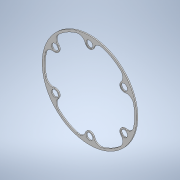
# Autodesk Inventor part: Bottom Lid
Saved by Autodesk Inventor 2020 (Build 240168000, 168)
## iProperties
Created: 2020-03-28
Part Number: Bottom Lid
Material: Generic
Document SubType Name: Modeling
Designer: pengpeng
Density: 1 g/cm^3
Appearance: Default
Author: pengpeng
Autodesk Inventor part; units mm, degrees
ref_plane "YZ Plane" through (0, 0, 0) normal (1, 0, 0) x (0, 1, 0)
ref_plane "XZ Plane" through (0, 0, 0) normal (0, 1, 0) x (-1, 0, 0)
ref_plane "XY Plane" through (0, 0, 0) normal (0, 0, 1) x (1, 0, 0)
sketch "Sketch1" plane through (0, 0, 0) normal (0, 0, 1) x (1, 0, 0)
  circle A0 centre (0, 0) radius 68
  circle A1 centre (0, 0) radius 65
  line L0 (0, 0) -> (0, 94.1006) construction
  line L1 (0, 0) -> (-100.1308, -57.8105) construction
  line L2 (0, 0) -> (108.5937, -62.6966) construction
  line L3 (0, 0) -> (0, -119.3862) construction
  line L4 (0, 0) -> (-99.0917, 57.2106) construction
  line L5 (0, 0) -> (100.283, 57.8984) construction
  circle A2 centre (0, 57.5) radius 4.8
  circle A3 centre (-49.7965, 28.75) radius 4.8
  circle A4 centre (-49.7965, -28.75) radius 4.8
  circle A5 centre (0, -57.5) radius 4.8
  circle A6 centre (49.7965, -28.75) radius 4.8
  circle A7 centre (49.7965, 28.75) radius 4.8
  circle A8 centre (0, 57.5) radius 6.3
  circle A9 centre (-49.7965, 28.75) radius 6.3
  circle A10 centre (-49.7965, -28.75) radius 6.3
  circle A11 centre (0, -57.5) radius 6.3
  circle A12 centre (49.7965, -28.75) radius 6.3
  circle A13 centre (49.7965, 28.75) radius 6.3
  circle A14 centre (-15.5907, 52.744) radius 10
  circle A15 centre (15.5907, 52.744) radius 10
  circle A16 centre (-53.473, 12.87) radius 10
  circle A17 centre (-37.8823, 39.874) radius 10
  circle A18 centre (-37.8823, -39.874) radius 10
  circle A19 centre (-53.473, -12.87) radius 10
  circle A20 centre (15.5907, -52.744) radius 10
  circle A21 centre (-15.5907, -52.744) radius 10
  circle A22 centre (53.473, -12.87) radius 10
  circle A23 centre (37.8823, -39.874) radius 10
  circle A24 centre (37.8823, 39.874) radius 10
  circle A25 centre (53.473, 12.87) radius 10
  point P0 (63.1954, 15.2101)
  point P1 (63.1954, -15.2101)
  point P2 (51.2175, -22.6123)
  point P3 (45.1916, -33.0494)
  point P4 (44.77, -47.1238)
  point P5 (18.4254, -62.3338)
  point P6 (6.0259, -55.6618)
  point P7 (-6.0259, -55.6618)
  point P8 (-18.4254, -62.3338)
  point P9 (-44.77, -47.1238)
  point P10 (-45.1916, -33.0494)
  point P11 (-51.2175, -22.6123)
  point P12 (-63.1954, -15.2101)
  point P13 (-63.1954, 15.2101)
  point P14 (-51.2175, 22.6123)
  point P15 (-45.1916, 33.0494)
  point P16 (-44.77, 47.1238)
  point P17 (-18.4254, 62.3338)
  point P18 (-6.0259, 55.6618)
  point P19 (6.0259, 55.6618)
  point P20 (18.4254, 62.3338)
  point P21 (44.77, 47.1238)
  point P22 (45.1916, 33.0494)
  point P23 (51.2175, 22.6123)
  dimension "d0" = 136
  dimension "d1" = 130
  dimension "d2" = 120
  dimension "d3" = 120
  dimension "d4" = 120
  dimension "d5" = 120
  dimension "d6" = 9.6
  dimension "d7" = 57.5
  dimension "d10" = 360
  dimension "d12" = 1.5
  dimension "d15" = 360
  dimension "d17" = 20
  dimension "d18" = 20
  dimension "d21" = 360
  constraints: 26 centre point, 12 end point, 4 tangent, 2 coincident, 2 point on line, 1 vertical, 51 other
  measures "d0" diameter of A0
  measures "d1" diameter of A1
  measures "d2" angle of L1 L0
  measures "d3" angle of L2 L1
  measures "d4" angle of L5 L4
  measures "d5" angle of L3 L5
  measures "d6" diameter of A2
  measures "d7" distance of L0.start A2.centre
  measures "d12" radial gap between concentric circles of A2 A8
  measures "d17" diameter of A14
  measures "d18" diameter of A15
extrude "Extrusion1" add sketch "Sketch1" along normal blind 1.5 contours A0 | A25 A13 A24 A1 | A1 A23 A12 A22 | A13 | A12 | A15 A8 A14 A1 | A1 A21 A11 A20 | A8 | A11 | A17 A9 A16 A1 | A1 A19 A10 A18 | A9 | A10
equation "\"d3\" = d2"
equation "\"d4\" = d2"
equation "\"d5\" = d4"
equation "\"d18\" = d17"
body "Solid1"
